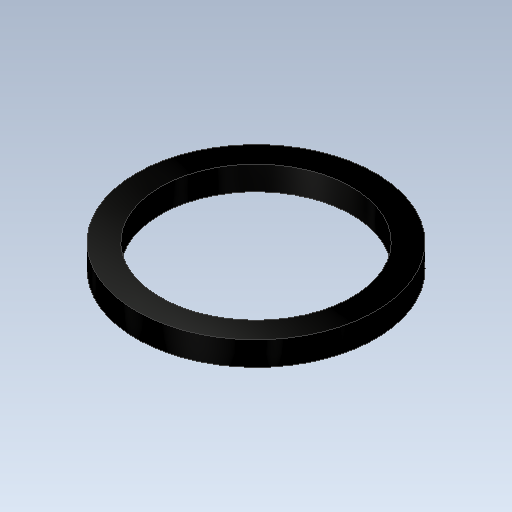
# Autodesk Inventor part: speed_washer
Saved by Autodesk Inventor 2020.1 (Build 241239000, 239)
## iProperties
Created: 2018-11-23
Part Number: speed_washer
Material: Aluminum 6061-AHC
Document SubType Name: Modeling
Designer: Petar
Density: 2.7 g/cm^3
Appearance: Aluminum Frame - Anodized Dark Bronze Satin
Mass: 0.0763407 g
Surface Area: 1.13097 cm^2
Volume: 0.0282743 cm^3
Author: Petar
Autodesk Inventor part; units mm, degrees
ref_plane "YZ Plane" through (0, 0, 0) normal (1, 0, 0) x (0, 1, 0)
ref_plane "XZ Plane" through (0, 0, 0) normal (0, 1, 0) x (-1, 0, 0)
ref_plane "XY Plane" through (0, 0, 0) normal (0, 0, 1) x (1, 0, 0)
sketch "Sketch1" plane through (0, 0, 0) normal (0, 1, 0) x (-1, 0, 0)
  circle A0 centre (0, 0) radius 4
  circle A1 centre (0, 0) radius 5
  dimension "d0" = 8
  dimension "d1" = 10
  constraints: 2 centre point, 2 coincident
  measures "d0" diameter of A0
  measures "d1" diameter of A1
extrude "Extrusion1" add sketch "Sketch1" along normal blind 1
body "Solid1"
